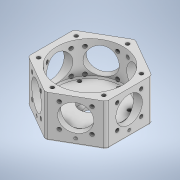
# Autodesk Inventor part: crankcase
Saved by Autodesk Inventor 2020 (Build 240168000, 168)
## iProperties
Created: 2020-08-05
Part Number: crankcase
Material: Generic
Document SubType Name: Modeling
Designer: benny
Density: 1 g/cm^3
Appearance: Default
Author: benny
Autodesk Inventor part; units mm, degrees
ref_plane "XZ Plane" through (0, 0, 0) normal (0, 1, 0) x (-1, 0, 0)
ref_plane "XY Plane" through (0, 0, 0) normal (0, 0, 1) x (1, 0, 0)
sketch "Sketch1" plane through (0, 0, 0) normal (0, 1, 0) x (-1, 0, 0)
  line L0 (0, -61.1991) -> (-53, -30.5996)
  line L1 (-53, -30.5996) -> (-53, 30.5996)
  line L2 (-53, 30.5996) -> (0, 61.1991)
  line L3 (0, 61.1991) -> (53, 30.5996)
  line L4 (53, 30.5996) -> (53, -30.5996)
  line L5 (53, -30.5996) -> (0, -61.1991)
  point P0 (0, 0)
  point P1 (0, 0)
  point P2 (26.5, -45.8993)
  dimension "d1" = 0
  dimension "d2" = 0
  constraints: 12 end point, 1 midpoint, 1 vertical, 13 other
  measures "d1" distance of point (0, 0) point (0, 0)
  measures "d2" distance of point (0, 0) point (0, 0)
extrude "Extrusion1" add sketch "Sketch1" along normal blind 57
sketch "Sketch2" plane through (0, 57, 0) normal (0, 1, 0) x (1, 0, 0)
  circle A0 centre (0, 0) radius 45
  dimension "d5" = 90
  constraints: 1 centre point, 1 coincident
  measures "d5" diameter of A0
extrude "Extrusion2" cut sketch "Sketch2" against normal blind 45
sketch "Sketch5" plane through (0, 0, 0) normal (0, 0, 1) x (1, 0, 0)
  line L0 (-45, 12) -> (45, 12) projected
  line L1 (45, 12) -> (45, 14)
  line L2 (45, 57) -> (45, 12) projected
  line L3 (44.3429, 12) -> (42.3429, 12)
  line L4 (42.3429, 12) -> (44.3429, 14)
  line L5 (44.3429, 14) -> (44.3429, 12)
  line L6 (0, -11.4) -> (0, 68.4) projected
  point P0 (0, 0)
  dimension "d11" = 2
  dimension "d12" = 2
  constraints: 8 end point, 3 point on line, 1 perpendicular
  measures "d11" distance of L0.end L1.end
  measures "d12" distance of L3.start L3.end
revolve "Revolution1" add sketch "Sketch5" angle 360 about axis through (0, -10, 0) along (0, 1, 0)
fillet "Fillet1" radius 5 6 edges at (-53, 28.5, -30.5996) (-53, 28.5, 30.5996) (0, 28.5, -61.1991) (53, 28.5, -30.5996) (0, 28.5, 61.1991) (53, 28.5, 30.5996)
fillet "Fillet2" radius 2 12 edges at (0, 0, 60.4256) (26.5, 0, 45.8993) (52.3301, 0, 30.2128) (53, 0, 0) (52.3301, 0, -30.2128) (26.5, 0, -45.8993) (0, 0, -60.4256) (-26.5, 0, -45.8993) (-52.3301, 0, -30.2128) (-53, 0, 0) (-52.3301, 0, 30.2128) (-26.5, 0, 45.8993)
sketch "Sketch6" plane through (0, 0, 0) normal (0, -1, 0) x (1, 0, 0)
  circle A0 centre (0, 0) radius 7
  dimension "d16" = 14
  constraints: 1 centre point, 1 coincident
  measures "d16" diameter of A0
extrude "Extrusion3" cut sketch "Sketch6" against normal blind 4
sketch "Sketch8" plane through (0, 12, 0) normal (0, 1, 0) x (1, 0, 0)
  circle A0 centre (0, 0) radius 7 projected
  circle A1 centre (0, 0) radius 14
  dimension "d22" = 28
  constraints: 1 centre point, 1 coincident
  measures "d22" diameter of A1
extrude "Extrusion5" cut sketch "Sketch8" against normal blind 8 contours A0 | A1
sketch "Sketch9" plane through (2.5, 2, -59.7558) normal (0.5, 0, -0.8660254) x (-0.8660254, 0, -0.5)
  line L0 (-72.7128, 55) -> (17.2872, 55) projected
  line L1 (-27.7128, 55) -> (-27.7128, 30)
  circle A0 centre (-27.7128, 30) radius 18
  point P0 (-27.7128, -2)
  dimension "d25" = 25
  dimension "d26" = 36
  constraints: 2 end point, 1 centre point, 1 coincident, 1 midpoint, 1 vertical
  measures "d25" distance of L1.start L1.end
  measures "d26" diameter of A0
extrude "Extrusion6" cut sketch "Sketch9" against normal blind 17.525
pattern_circular "Circular Pattern1" count 6 over 360 about axis through (0, 57, 0) along (0, -1, 0) of "Extrusion6"
sketch "Sketch10" plane through (0, 57, 0) normal (0, 1, 0) x (1, 0, 0)
  circle A0 centre (0, 0) radius 7 projected
  line L0 (0, 0) -> (0, 51)
  dimension "d32" = 51
  constraints: 2 end point, 1 vertical
  measures "d32" distance of L0.start L0.end
hole "Hole1" at (0, 57, -51) direction (0, -1, 0) diameter 4.917 depth 17.1 tip angle 118 thread size "M6x1" class "6H" standard "ISO Metric profile"
pattern_circular "Circular Pattern2" count 6 over 360 about axis through (0, 57, 0) along (0, -1, 0) of "Hole1"
ref_plane "Work Plane1" through (0, 8, 0) normal (0, -1, 0) x (1, 0, 0)
sketch "Sketch14" plane through (-53, 57, -27.7128) normal (-1, 0, 0) x (0, 0, 1)
  circle A0 centre (27.7128, -49) radius 2
  point P0 (27.7128, -57)
  dimension "d52" = 4
  constraints: 1 centre point
  measures "d52" diameter of A0
extrude "Extrusion8" cut sketch "Sketch14" against normal blind 36
sketch "Sketch16" plane through (0, 0, 0) normal (0, -1, 0) x (1, 0, 0)
  line L0 (0, 0) -> (-20, 0)
  circle A0 centre (-20, 0) radius 2
  dimension "d56" = 20
  dimension "d57" = 4
  constraints: 2 end point, 1 centre point, 1 coincident, 1 horizontal
  measures "d56" distance of L0.start L0.end
  measures "d57" diameter of A0
extrude "Extrusion9" cut sketch "Sketch16" against normal blind 8
pattern_circular "Circular Pattern4" count 6 over 360 about axis through (0, 0, 0) along (0, 1, 0) of "Extrusion8", "Extrusion9"
sketch "Sketch17" plane through (0, 0, 0) normal (0, -1, 0) x (1, 0, 0)
  line L0 (0, 0) -> (0, 39)
  dimension "d63" = 39
  constraints: 2 end point, 1 vertical
  measures "d63" distance of L0.start L0.end
hole "Hole2" at (0, 0, 39) direction (0, 1, 0) diameter 4.917 depth 17.1 tip angle 118 thread size "M6x1" class "6H" standard "ISO Metric profile"
pattern_circular "Circular Pattern5" count 6 over 360 about axis through (0, 0, 0) along (0, 1, 0) of "Hole2"
ref_plane "Work Plane2" through (53, 0, 0) normal (1, 0, 0) x (0, 1, 0)
sketch "Sketch20" plane through (53, 57, 27.7128) normal (1, 0, 0) x (0, 0, -1)
  circle A0 centre (27.7128, -25) radius 18 projected
  line L0 (27.7128, -25) -> (43.9763, -41.2635)
  line L1 (27.7128, -25) -> (50.7128, -25) construction
  point P0 (27.7128, -57)
  dimension "d75" = 23
  dimension "d76" = 45
  constraints: 4 end point, 1 equal length, 1 horizontal
  measures "d75" distance of L0.start L0.end
  measures "d76" angle of L0 L1
hole "Hole3" at (53, 15.7365, -16.2635) direction (-1, 0, 0) diameter 4.917 depth 17.1 tip angle 118 thread size "M6x1" class "6H" standard "ISO Metric profile"
pattern_circular "Circular Pattern6" count 4 over 360 about axis through (53, 32, 0) along (-1, 0, 0) of "Hole3"
pattern_circular "Circular Pattern7" count 6 over 360 about axis through (0, 0, 0) along (0, 1, 0) of "Hole3", "Circular Pattern6"
body "Solid1"
